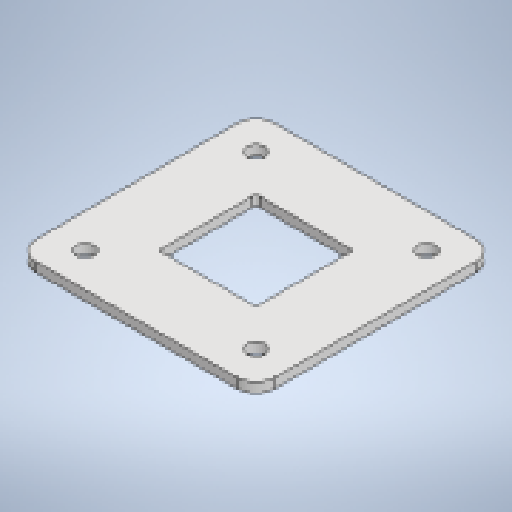
# Autodesk Inventor part: ANP 1425 FDS Way FLANGE
Saved by Autodesk Inventor 2025.3 (Build 293356030, 356C)
## iProperties
Created: 2025-06-24
Part Number: ANP 1425 FDS Way FLANGE
Material: Stainless Steel
Document SubType Name: Sheet Metal
Designer: user
Mass: 82.1885 g
Surface Area: 82.7314 cm^2
Volume: 10.2736 cm^3
Density: 8 g/cm^3
Sheet Metal Rule: AISI304 2mm Die16
Sheet Metal Width: 74,200 mm
Sheet Metal Length: 74,200 mm
Sheet Metal Area: 5505,640 mm^2
Appearance: Default
Flat Pattern Width: 7.42 cm
Flat Pattern Length: 7.42 cm
Flat Pattern Area: 55.0564 cm^2
Author: user
Autodesk Inventor part; units mm, degrees
ref_plane "YZ Plane" through (0, 0, 0) normal (1, 0, 0) x (0, 1, 0)
ref_plane "XZ Plane" through (0, 0, 0) normal (0, 1, 0) x (-1, 0, 0)
ref_plane "XY Plane" through (0, 0, 0) normal (0, 0, 1) x (1, 0, 0)
sketch "Sketch1" plane through (0, 0, 0) normal (0, 0, 1) x (1, 0, 0)
  line L0 (-37.1, -37.1) -> (37.1, -37.1)
  line L1 (37.1, -37.1) -> (37.1, 37.1)
  line L2 (37.1, 37.1) -> (-37.1, 37.1)
  line L3 (-37.1, 37.1) -> (-37.1, -37.1)
  line L4 (-37.1, -37.1) -> (37.1, 37.1) construction
  line L5 (37.1, -37.1) -> (-37.1, 37.1) construction
  line L6 (15.1, -15.1) -> (-15.1, -15.1)
  line L7 (-15.1, -15.1) -> (-15.1, 15.1)
  line L8 (-15.1, 15.1) -> (15.1, 15.1)
  line L9 (15.1, 15.1) -> (15.1, -15.1)
  line L10 (15.1, -15.1) -> (-15.1, 15.1) construction
  line L11 (-15.1, -15.1) -> (15.1, 15.1) construction
  point P0 (0, 0)
  dimension "d172" = 30.2
  dimension "d181" = 22
  dimension "d187" = 22
  measures "d172" distance of L7.end L8.end
  measures "d181" distance between parallel lines of L1 L9
  measures "d187" distance between parallel lines of L2 L8
extrude "Plate5" add sketch "Sketch1" along normal blind 3
sketch "Sketch9" plane through (0, 0, 3) normal (0, 0, 1) x (1, 0, 0)
  circle A0 centre (26.5165, -26.5165) radius 2.75
  line L0 (26.5165, 26.5165) -> (-26.5165, 26.5165) construction
  line L1 (-26.5165, 26.5165) -> (-26.5165, -26.5165) construction
  line L2 (-26.5165, -26.5165) -> (26.5165, -26.5165) construction
  line L3 (26.5165, -26.5165) -> (26.5165, 26.5165) construction
  line L4 (26.5165, 26.5165) -> (-26.5165, -26.5165) construction
  line L5 (-26.5165, 26.5165) -> (26.5165, -26.5165) construction
  circle A1 centre (-26.5165, -26.5165) radius 2.75
  circle A2 centre (26.5165, 26.5165) radius 2.75
  circle A3 centre (-26.5165, 26.5165) radius 2.75
  circle A4 centre (0, 0) radius 37.5 construction
  line L6 (-15.1, -15.1) -> (-15.1, 15.1) projected
  line L7 (-15.1, 15.1) -> (15.1, 15.1) projected
  line L8 (15.1, 15.1) -> (15.1, -15.1) projected
  line L9 (15.1, -15.1) -> (-15.1, -15.1) projected
  line L10 (37.1, -37.1) -> (-37.1, -37.1) projected
  line L11 (37.1, 37.1) -> (37.1, -37.1) projected
  line L12 (-37.1, 37.1) -> (37.1, 37.1) projected
  line L13 (-37.1, -37.1) -> (-37.1, 37.1) projected
  line L14 (-15, 15) -> (15, 15) construction
  line L15 (15, 15) -> (15, -15) construction
  line L16 (15, -15) -> (-15, -15) construction
  line L17 (-15, -15) -> (-15, 15) construction
  line L18 (-15, -15) -> (15, 15) construction
  dimension "d188" = 75
  dimension "d174" = 5.5
  dimension "d184" = 30
  dimension "d185" = 30
  dimension "d186" = 16.2868
  constraints: 22 end point, 8 coincident, 4 centre point, 4 parallel, 3 equal radius, 3 midpoint, 3 perpendicular, 2 horizontal, 3 other
  measures "d174" diameter of A0
  measures "d184" distance of L14.start L14.end
  measures "d185" distance of L14.end L15.end
  measures "d186" distance of L0.end L14.start
extrude "Cut2" cut sketch "Sketch9" against normal blind 3 contours A0 | A1 | A2 | A3
fillet "Corner Round1" radius 6 4 edges at (37.1, 37.1, 1.5) (-37.1, 37.1, 1.5) (-37.1, -37.1, 1.5) (37.1, -37.1, 1.5)
fillet "Corner Round2" radius 1 4 edges at (-15.1, 15.1, 1.5) (-15.1, -15.1, 1.5) (15.1, -15.1, 1.5) (15.1, 15.1, 1.5)
body "Solid3"
